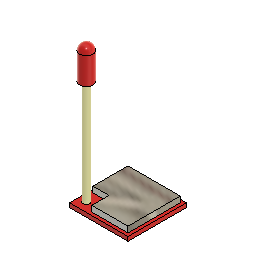
TWE-Lite-RED (Autodesk Fusion 360 design; units mm, degrees)
Autodesk Fusion 360 part; units mm, degrees
sketch "スケッチ1" plane through (0, 0, 0) normal (0, 0, 1) x (1, 0, 0)
  line L0 (6.985, -6.985) -> (-6.985, -6.985)
  line L1 (-6.985, -6.985) -> (-6.985, 6.985)
  line L2 (-6.985, 6.985) -> (6.985, 6.985)
  line L3 (6.985, 6.985) -> (6.985, -6.985)
  line L4 (6.985, -6.985) -> (-6.985, 6.985) construction
  line L5 (-6.985, -6.985) -> (6.985, 6.985) construction
  dimension "d1" = 13.97
  dimension "d2" = 13.97
  constraint horizontal L0
  constraint perpendicular L0 L1
  constraint parallel L0 L2
  constraint parallel L1 L3
  constraint coincident L4 origin
  constraint coincident L5 origin
  measures "d1" distance of L1.end L2.end
  measures "d2" distance of L0.end L1.end
extrude "押し出し1" add sketch "スケッチ1" along normal blind 1 makes body 1
sketch "スケッチ2" plane through (0, 0, 1) normal (0, 0, 1) x (-1, 0, 0)
  line L0 (-6.985, -6.985) -> (6.985, -6.985)
  line L1 (6.985, -6.985) -> (6.985, 6.985)
  line L2 (6.985, 6.985) -> (-6.985, 6.985)
  line L3 (-6.985, 6.985) -> (-6.985, -6.985)
  line L4 (-6.25, -6.25) -> (6.25, -6.25)
  line L5 (6.25, -6.25) -> (6.25, 6.25)
  line L6 (6.25, 6.25) -> (-6.25, 6.25)
  line L7 (-6.25, 6.25) -> (-6.25, -6.25)
  line L8 (-6.25, -6.25) -> (6.25, 6.25) construction
  line L9 (6.25, -6.25) -> (-6.25, 6.25) construction
  circle A0 centre (5.185, 4.785) radius 0.45
  line L10 (6.25, -6.25) -> (6.25, 2.15)
  line L11 (-6.25, 6.25) -> (2.4, 6.25)
  line L12 (2.4, 6.25) -> (2.4, 2.15)
  line L13 (2.4, 2.15) -> (6.25, 2.15)
  dimension "d20" = 12.5
  dimension "d21" = 12.5
  dimension "d24" = 0.9
  dimension "d25" = 8.4
  dimension "d26" = 8.65
  constraint horizontal L4
  constraint perpendicular L4 L5
  constraint parallel L4 L6
  constraint parallel L5 L7
  constraint coincident L8 origin
  constraint coincident L9 origin
  constraint perpendicular L4 L10
  constraint perpendicular L7 L11
  constraint perpendicular L11 L12
  constraint perpendicular L5 L13
  measures "d20" distance of L5.end L6.end
  measures "d21" distance of L4.end L5.end
  measures "d24" diameter of A0
  measures "d25" distance of L4.end L10.end
  measures "d26" distance of L6.end L11.end
extrude "押し出し2" add sketch "スケッチ2" along normal blind 1.4 separate body contours L4 L5 L6 L7 L10 L11 L12 L13 makes body 2
extrude "押し出し3" cut sketch "スケッチ2" against normal blind 1 contours A0 bodies 1
cylinder "円柱プリミティブ1" add diameter 0.8 height 2 placed x (1, 0, 0) y (0, 1, 0) z (0, 0, 1) at (11, 0, 0) separate body makes body 3
cylinder "円柱プリミティブ2" add diameter 1.6 height 25 placed x (1, 0, 0) y (0, 1, 0) z (0, 0, 1) at (11, 0, 2) bodies 3
cylinder "円柱プリミティブ3" add diameter 3.2 height 8 placed x (1, 0, 0) y (0, 1, 0) z (0, 0, 1) at (11, 0, 27) bodies 3
fillet "フィレット1" radius 1.6 1 edges at (9.5083, -0.5786, 35) on bodies 3
copy_body "ボディ -> コンポーネント1" bodies 3 removing the originals makes body 4 in component "アンテナ"
component "アンテナ" placed x (1, 0, 0) y (0, 1, 0) z (0, 0, 1) at (-16.185, -4.785, -1)
